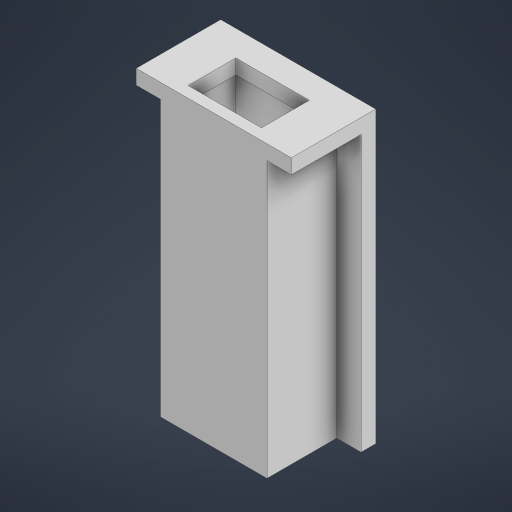
# Autodesk Inventor part: UE306_Sleeve
Saved by Autodesk Inventor 2023 (Build 270158000, 158)
## iProperties
Created: 2023-02-13
Part Number: UE306_Sleeve
Material: Generic
Document SubType Name: Modeling
Designer: uzair
Density: 1 g/cm^3
Appearance: Default
Author: uzair
Autodesk Inventor part; units mm, degrees
ref_plane "YZ Plane" through (0, 0, 0) normal (1, 0, 0) x (0, 1, 0)
ref_plane "XZ Plane" through (0, 0, 0) normal (0, 1, 0) x (-1, 0, 0)
ref_plane "XY Plane" through (0, 0, 0) normal (0, 0, 1) x (1, 0, 0)
sketch "Sketch1" plane through (0, 0, 0) normal (0, 1, 0) x (-1, 0, 0)
  line L0 (36.83, 24.13) -> (-36.83, 24.13)
  line L1 (-36.83, 24.13) -> (-36.83, -24.13)
  line L2 (-36.83, -24.13) -> (36.83, -24.13)
  line L3 (36.83, -24.13) -> (36.83, 24.13)
  line L4 (36.83, 24.13) -> (-36.83, -24.13) construction
  line L5 (-36.83, 24.13) -> (36.83, -24.13) construction
  line L6 (29.21, 20.32) -> (-29.21, 20.32)
  line L7 (-29.21, 20.32) -> (-29.21, -20.32)
  line L8 (-29.21, -20.32) -> (29.21, -20.32)
  line L9 (29.21, -20.32) -> (29.21, 20.32)
  line L10 (29.21, 20.32) -> (-29.21, -20.32) construction
  line L11 (-29.21, 20.32) -> (29.21, -20.32) construction
  point P0 (0, 0)
  dimension "d0" = 73.66
  dimension "d1" = 48.26
  dimension "d2" = 58.42
  dimension "d3" = 40.64
  constraints: 24 end point, 4 midpoint, 4 parallel, 2 horizontal, 2 perpendicular
  measures "d0" distance of L2.end L1.end
  measures "d1" distance of L1.end L0.end
  measures "d2" distance of L8.end L7.end
  measures "d3" distance of L7.end L6.end
extrude "Extrusion1" add sketch "Sketch1" along normal blind 190.5
sketch "Sketch2" plane through (36.83, 0, 24.13) normal (1, 0, 0) x (0, 0, -1)
  line L0 (0, 0) -> (-10.16, 0)
  line L1 (48.26, 0) -> (48.26, 190.5) projected
  line L2 (48.26, 0) -> (58.42, 0)
  line L3 (-10.16, 0) -> (58.42, 0)
  line L4 (58.42, 0) -> (58.42, 190.5)
  line L5 (58.42, 190.5) -> (-10.16, 190.5)
  line L6 (-10.16, 190.5) -> (-10.16, 0)
  line L7 (-10.16, 190.5) -> (58.42, 190.5)
  line L8 (58.42, 190.5) -> (58.42, 200.66)
  line L9 (58.42, 200.66) -> (-10.16, 200.66)
  line L10 (-10.16, 200.66) -> (-10.16, 190.5)
  line L11 (0, 190.5) -> (48.26, 190.5) projected
  line L12 (-10.16, 0) -> (0, 0)
  line L13 (0, 0) -> (0, 190.5)
  line L14 (0, 190.5) -> (-10.16, 190.5)
  line L15 (-10.16, 190.5) -> (-10.16, 0)
  line L16 (0, 190.5) -> (58.42, 190.5)
  line L17 (58.42, 190.5) -> (58.42, 200.66)
  line L18 (58.42, 200.66) -> (0, 200.66)
  line L19 (0, 200.66) -> (0, 190.5)
  point P0 (24.13, 0)
  dimension "d6" = 10.16
  dimension "d7" = 10.16
  dimension "d8" = 10.16
  constraints: 36 end point, 8 parallel, 6 horizontal, 4 perpendicular
  measures "d6" distance of L0.start L0.end
  measures "d7" distance of L1.start L2.end
  measures "d8" distance of L8.end L7.end
extrude "Extrusion2" add sketch "Sketch2" against normal blind 90.5129 contours L1 L5 L4 L2 | L19 L9 L8 L5
extrude "Extrusion3" add sketch "Sketch2" along normal blind 16.8529 contours L1 L5 L4 L2 | L19 L9 L8 L5
sketch "Sketch3" plane through (-29.21, 190.5, 20.32) normal (0, -1, 0) x (1, 0, 0)
  line L0 (58.42, 0) -> (0, 0) projected
  line L1 (0, -40.64) -> (58.42, -40.64) projected
  line L2 (58.42, 0) -> (0, 0)
  line L3 (0, 0) -> (0, -40.64)
  line L4 (0, -40.64) -> (58.42, -40.64)
  line L5 (58.42, -40.64) -> (58.42, 0)
  line L6 (54.61, -3.81) -> (3.81, -3.81)
  line L7 (3.81, -3.81) -> (3.81, -36.83)
  line L8 (3.81, -36.83) -> (54.61, -36.83)
  line L9 (54.61, -36.83) -> (54.61, -3.81)
  line L10 (54.61, -3.81) -> (3.81, -36.83) construction
  line L11 (3.81, -3.81) -> (54.61, -36.83) construction
  point P0 (29.21, -20.32)
  dimension "d13" = 50.8
  dimension "d14" = 33.02
  constraints: 20 end point, 4 parallel, 2 horizontal, 2 midpoint, 2 perpendicular
  measures "d13" distance of L8.end L7.end
  measures "d14" distance of L7.end L6.end
extrude "Extrusion4" cut sketch "Sketch3" against normal blind 10.16 contours L9 L8 L7 L6
body "Solid1"
